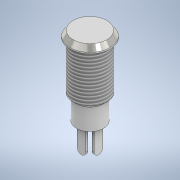
# Autodesk Inventor part: LED Indicator Farnell 19100054
Saved by Autodesk Inventor 2021 (Build 250183000, 183)
## iProperties
Created: 2020-07-20
Part Number: LED Indicator Farnell 19100054
Material: Generic
Document SubType Name: Modeling
Designer: jgray
Density: 1 g/cm^3
Appearance: Default
Author: jgray
Autodesk Inventor part; units mm, degrees
ref_plane "YZ Plane" through (0, 0, 0) normal (1, 0, 0) x (0, 1, 0)
ref_plane "XZ Plane" through (0, 0, 0) normal (0, 1, 0) x (-1, 0, 0)
ref_plane "XY Plane" through (0, 0, 0) normal (0, 0, 1) x (1, 0, 0)
sketch "Sketch1" plane through (0, 0, 0) normal (0, 1, 0) x (-1, 0, 0)
  circle A0 centre (0, 0) radius 4.75
  dimension "d0" = 9.5
  constraints: 1 centre point, 1 coincident
  measures "d0" diameter of A0
extrude "Extrusion1" add sketch "Sketch1" along normal blind 1.5
chamfer "Chamfer1" distance 0.8 distance2 1.2 1 edges at (4.75, 1.5, 0) measured on face at (-1.1851, 1.5, -1.0499)
sketch "Sketch2" plane through (0, 0, 0) normal (0, -1, 0) x (1, 0, 0)
  circle A0 centre (0, 0) radius 4
  dimension "d6" = 8
  constraints: 1 centre point, 1 coincident
  measures "d6" diameter of A0
extrude "Extrusion2" add sketch "Sketch2" along normal blind 12
chamfer "Chamfer2" distance 0.8 angle 45 1 edges at (-4, -12, 0)
thread "Thread1" size "M8x0.75" class "6g" standard "ANSI Metric M Profile" length 12.5
sketch "Sketch3" plane through (0, -12, 0) normal (0, -1, 0) x (1, 0, 0)
  circle A0 centre (0, 0) radius 3.2
  constraints: 1 centre point, 1 coincident
extrude "Extrusion3" add sketch "Sketch3" along normal blind 5
sketch "Sketch4" plane through (0, -17, 0) normal (0, -1, 0) x (1, 0, 0)
  line L0 (1.75, -1.75) -> (-1.75, -1.75)
  line L1 (1.75, -1.75) -> (-1.75, 1.75) construction
  line L2 (-1.75, -1.75) -> (1.75, 1.75) construction
  line L3 (0, 6.1884) -> (0, -7.5413) construction
  line L4 (-9.3951, 0) -> (6.4878, 0) construction
  line L5 (1, 1.5) -> (-1, 1.5)
  line L6 (-1, 1.5) -> (-1, 2)
  line L7 (-1, 2) -> (1, 2)
  line L8 (1, 2) -> (1, 1.5)
  line L9 (1, 1.5) -> (-1, 2) construction
  line L10 (-1, 1.5) -> (1, 2) construction
  line L11 (2, -1) -> (1.5, -1)
  line L12 (1.5, -1) -> (1.5, 1)
  line L13 (1.5, 1) -> (2, 1)
  line L14 (2, 1) -> (2, -1)
  line L15 (2, -1) -> (1.5, 1) construction
  line L16 (1.5, -1) -> (2, 1) construction
  line L17 (-1.5, -1) -> (-2, -1)
  line L18 (-2, -1) -> (-2, 1)
  line L19 (-2, 1) -> (-1.5, 1)
  line L20 (-1.5, 1) -> (-1.5, -1)
  line L21 (-1.5, -1) -> (-2, 1) construction
  line L22 (-2, -1) -> (-1.5, 1) construction
  line L23 (1.75, 1.75) -> (1.75, 1)
  line L24 (1.75, -1) -> (1.75, -1.75)
  line L25 (-1.75, -1.75) -> (-1.75, -1)
  line L26 (-1.75, 1) -> (-1.75, 1.75)
  line L27 (-1.75, 1.75) -> (-1, 1.75)
  line L28 (1, 1.75) -> (1.75, 1.75)
  point P0 (0, 0)
  point P1 (0, 0)
  point P2 (0, 0)
  dimension "d16" = 3.5
  dimension "d17" = 3.5
  dimension "d18" = 2
  dimension "d19" = 0.5
  dimension "d20" = 0.5
  dimension "d21" = 2
  dimension "d22" = 0.5
  dimension "d23" = 2
  constraints: 58 end point, 12 parallel, 10 midpoint, 5 horizontal, 5 perpendicular, 2 point on line, 1 vertical
  measures "d16" distance of L1.end L2.end
  measures "d17" distance of L0.end L1.end
  measures "d18" distance of L6.end L7.end
  measures "d19" distance of L5.end L6.end
  measures "d20" distance of L12.end L13.end
  measures "d21" distance of L11.end L12.end
  measures "d22" distance of L18.end L19.end
  measures "d23" distance of L17.end L18.end
extrude "Extrusion4" add sketch "Sketch4" along normal blind 6 contours L11 L12 L13 L14 | L17 L18 L19 L20 | L8 L5 L6 L7
fillet "Fillet1" radius 1 6 edges at (-1.75, -23, 1) (-1.75, -23, -1) (-1, -23, 1.75) (1, -23, 1.75) (1.75, -23, 1) (1.75, -23, -1)
body "Solid1"
